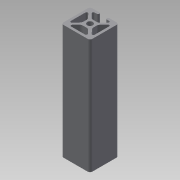
# Autodesk Inventor part: 25-2501
Saved by Autodesk Inventor 2013 (Build 170138000, 138)
## iProperties
Created: 2014-04-23
Part Number: 25-2501
Material: Generic
Document SubType Name: Modeling
Designer: Ross Bowman
Density: 1 g/cm^3
Engineer: Ross Bowman
Catalog Web Link: 8020.net
Vendor: 80/20 Inc.
Company: 80/20 Inc.
Author: Ross Bowman
Keywords: 80/20 , 8020 , T-Slot , Extrusion
Material: 6105-T5 Aluminum
Autodesk Inventor part; units mm, degrees
ref_plane "YZ Plane" through (0, 0, 0) normal (1, 0, 0) x (0, 1, 0)
ref_plane "XZ Plane" through (0, 0, 0) normal (0, 1, 0) x (-1, 0, 0)
ref_plane "XY Plane" through (0, 0, 0) normal (0, 0, 1) x (1, 0, 0)
sketch "Sketch1" plane through (0, 0, 0) normal (0, 0, 1) x (1, 0, 0)
  arc A0 (3.9004, -5.517) -> (1.5898, -4.52) centre (1.5898, -7.6958) ccw
  line L0 (6.8514, -8.6465) -> (3.9004, -5.517)
  arc A1 (6.1121, -10.36) -> (6.8514, -8.6465) centre (6.1121, -9.3437) ccw
  line L1 (-6.1121, -10.36) -> (6.1121, -10.36)
  arc A2 (-6.8514, -8.6465) -> (-6.1121, -10.36) centre (-6.1121, -9.3437) ccw
  line L2 (-3.9004, -5.517) -> (-6.8514, -8.6465)
  arc A3 (-1.5898, -4.52) -> (-3.9004, -5.517) centre (-1.5898, -7.6958) ccw
  line L3 (1.5898, -4.52) -> (-1.5898, -4.52)
  arc A4 (-10.36, -6.3382) -> (-8.5738, -7.0738) centre (-9.3466, -6.4137) ccw
  line L4 (-10.36, 6.3382) -> (-10.36, -6.3382)
  arc A5 (-8.5738, 7.0738) -> (-10.36, 6.3382) centre (-9.3466, 6.4137) ccw
  line L5 (-5.4693, 3.7815) -> (-8.5738, 7.0738)
  arc A6 (-4.38, 1.5898) -> (-5.4693, 3.7815) centre (-7.549, 1.3814) ccw
  line L6 (-4.38, -1.5898) -> (-4.38, 1.5898)
  arc A7 (-5.4693, -3.7815) -> (-4.38, -1.5898) centre (-7.549, -1.3814) ccw
  line L7 (-8.5738, -7.0738) -> (-5.4693, -3.7815)
  arc A8 (8.5693, -7.069) -> (10.36, -6.3423) centre (9.3463, -6.4139) ccw
  line L8 (5.2366, -3.5348) -> (8.5693, -7.069)
  arc A9 (4.38, -1.5898) -> (5.2366, -3.5348) centre (7.5472, -1.356) ccw
  line L9 (4.38, 1.5898) -> (4.38, -1.5898)
  arc A10 (5.2366, 3.5348) -> (4.38, 1.5898) centre (7.5472, 1.356) ccw
  line L10 (8.5693, 7.069) -> (5.2366, 3.5348)
  arc A11 (10.36, 6.3423) -> (8.5693, 7.069) centre (9.3463, 6.4139) ccw
  line L11 (10.36, -6.3423) -> (10.36, 6.3423)
  circle A12 centre (0, 0) radius 2.5
  arc A13 (-4.32, 10.36) -> (-4.32, 12.5) centre (-4.32, 11.43) ccw
  line L12 (-4.32, 12.5) -> (-10.5183, 12.5)
  arc A14 (-10.5183, 12.5) -> (-12.5, 10.5183) centre (-10.5183, 10.5183) ccw
  line L13 (-12.5, 10.5183) -> (-12.5, -10.5215)
  arc A15 (-12.5, -10.5215) -> (-10.6304, -12.5) centre (-10.5183, -10.5215) ccw
  line L14 (-10.6304, -12.5) -> (10.6304, -12.5)
  arc A16 (10.6304, -12.5) -> (12.5, -10.5215) centre (10.5183, -10.5215) ccw
  line L15 (12.5, -10.5215) -> (12.5, 10.5183)
  arc A17 (12.5, 10.5183) -> (10.5183, 12.5) centre (10.5183, 10.5183) ccw
  line L16 (10.5183, 12.5) -> (4.32, 12.5)
  arc A18 (4.32, 12.5) -> (4.32, 10.36) centre (4.32, 11.43) ccw
  line L17 (4.32, 10.36) -> (6.3685, 10.36)
  arc A19 (7.1102, 8.641) -> (6.3685, 10.36) centre (6.3685, 9.3405) ccw
  line L18 (7.1102, 8.641) -> (3.9004, 5.237)
  arc A20 (1.5898, 4.24) -> (3.9004, 5.237) centre (1.5898, 7.4158) ccw
  line L19 (1.5898, 4.24) -> (-1.5898, 4.24)
  arc A21 (-3.9004, 5.237) -> (-1.5898, 4.24) centre (-1.5898, 7.4158) ccw
  line L20 (-3.9004, 5.237) -> (-7.1102, 8.641)
  arc A22 (-6.3685, 10.36) -> (-7.1102, 8.641) centre (-6.3685, 9.3405) ccw
  line L21 (-6.3685, 10.36) -> (-4.32, 10.36)
  constraints: 44 end point, 44 point on circle, 23 centre point
extrude "Extrusion1" add sketch "Sketch1" against normal blind 100
body "Solid1"
